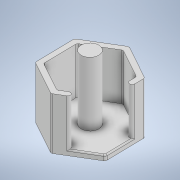
# Autodesk Inventor part: nicoles part
Saved by Autodesk Inventor 2020 (Build 240168000, 168)
## iProperties
Created: 2020-02-15
Part Number: nicoles part
Material: Generic
Document SubType Name: Modeling
Designer: jackm
Density: 1 g/cm^3
Appearance: Default
Author: jackm
Autodesk Inventor part; units mm, degrees
ref_plane "YZ Plane" through (0, 0, 0) normal (1, 0, 0) x (0, 1, 0)
ref_plane "XZ Plane" through (0, 0, 0) normal (0, 1, 0) x (-1, 0, 0)
ref_plane "XY Plane" through (0, 0, 0) normal (0, 0, 1) x (1, 0, 0)
sketch "Sketch2" plane through (0, 0, 0) normal (0, 1, 0) x (-1, 0, 0)
  line L0 (51.3491, -28.357) -> (1.1167, -58.6482)
  line L1 (1.1167, -58.6482) -> (-50.2324, -30.2912)
  line L2 (-50.2324, -30.2912) -> (-51.3491, 28.357)
  line L3 (-51.3491, 28.357) -> (-1.1167, 58.6482)
  line L4 (-1.1167, 58.6482) -> (50.2324, 30.2912)
  line L5 (50.2324, 30.2912) -> (51.3491, -28.357)
  point P0 (0, 0)
  point P1 (0, 0)
  dimension "d0" = 50.8
  constraints: 12 end point, 1 coincident, 13 other
  measures "d0" distance from line of L5 point (0, 0)
extrude "Extrusion1" add sketch "Sketch2" along normal blind 76.2
sketch "Sketch3" plane through (0, 76.2, 0) normal (0, 1, 0) x (1, 0, 0)
  line L0 (-42.6976, -25.7475) -> (-43.6468, 24.1034)
  line L1 (-43.6468, 24.1034) -> (-0.9492, 49.8509)
  line L2 (-0.9492, 49.8509) -> (42.6976, 25.7475)
  line L3 (42.6976, 25.7475) -> (42.9394, 13.0475)
  line L4 (13.6492, -42.1926) -> (0.9492, -49.8509)
  line L5 (0.9492, -49.8509) -> (-42.6976, -25.7475)
  line L6 (-50.2324, -30.2912) -> (1.1167, -58.6482) projected
  line L7 (13.6492, -42.1926) -> (46.2855, -59.4975)
  line L8 (46.2855, -59.4975) -> (75.5757, -4.2574)
  line L9 (75.5757, -4.2574) -> (42.9394, 13.0475)
  point P0 (0, 0)
  point P1 (0, 0)
  dimension "d3" = 180
  dimension "d4" = 43.18
  constraints: 18 end point, 1 coincident, 1 parallel, 11 other
  measures "d3" angle of L5 L6
  measures "d4" distance from line of L2 point (0, 0)
extrude "Extrusion2" cut sketch "Sketch3" against normal blind 68.58
fillet "Fillet1" radius 3.81 4 edges at (50.6385, 41.91, -8.9652) (21.5011, 41.91, 46.3559) (42.9394, 41.91, -13.0475) (13.6492, 41.91, 42.1926)
fillet "Fillet2" radius 1.905 4 edges at (50.9938, 7.62, 9.6959) (50.5769, 7.62, -12.2001) (18.6193, 7.62, 48.0938) (36.4251, 7.62, 37.3565)
sketch "Sketch4" plane through (0, 7.62, 0) normal (0, 1, 0) x (1, 0, 0)
  circle A0 centre (0, 0) radius 12.954
  dimension "d11" = 25.908
  constraints: 1 centre point, 1 coincident
  measures "d11" diameter of A0
extrude "Extrusion3" add sketch "Sketch4" along normal blind 93.98
fillet "Fillet3" radius 3.81 7 edges at (1.1167, 38.1, 58.6482) (-50.2324, 38.1, 30.2912) (-51.3491, 38.1, -28.357) (-1.1167, 38.1, -58.6482) (50.2324, 38.1, -30.2912) (50.7852, 7.062, 28.0455) (51.3491, 2.8575, 28.357)
fillet "Fillet4" radius 3.81 5 edges at (0.9492, 41.91, 49.8509) (42.6976, 41.91, -25.7475) (-0.9492, 41.91, -49.8509) (-43.6468, 41.91, -24.1034) (-42.6976, 41.91, 25.7475)
body "Solid1"
